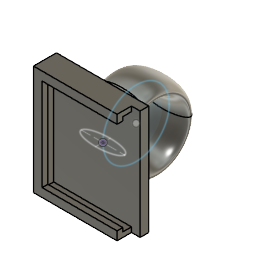
JoystickRingM1 (Autodesk Fusion 360 design; units mm, degrees)
part number: 2026-01-29-20-05-59-741
Autodesk Fusion 360 part; units mm, degrees
sketch "Sketch1" plane through (0, 0, 0) normal (0, 0, 1) x (1, 0, 0)
  ellipse E0 centre (0, 0) end of major axis (7.5, 0) minor radius 2.5
  line L0 (-7.5, 0) -> (7.5, 0) construction
  line L1 (0, -2.5) -> (0, 2.5) construction
  dimension "d1" = 15
  dimension "d2" = 5
  constraint coincident E0 L0.start
  constraint coincident E0 L0.end
  constraint coincident E0 L1.start
  constraint coincident E0 L1.end
  constraint coincident E0.centre origin
  constraint horizontal L0
  measures "d1" distance of E0
sketch "Sketch2" plane through (0, 0, 0) normal (1, 0, 0) x (0, 1, 0)
  circle A0 centre (11.5, 0) radius 11.5
  dimension "d4" = 23
  constraint coincident origin A0
  measures "d4" diameter of A0
sweep "Sweep1" add profiles "Sketch1" path "Sketch2" along A0 section 1 makes body 1
sketch "Sketch3" plane through (0, 0, 0) normal (1, 0, 0) x (0, 1, 0)
  line L0 (-0.1, -17.3) -> (-3.1, -17.3)
  line L1 (-3.1, -17.3) -> (-3.1, 17.3)
  line L2 (-3.1, 17.3) -> (-0.1, 17.3)
  line L3 (-0.1, 17.3) -> (-0.1, -17.3)
  dimension "d16" = 34.6
  dimension "d17" = 3
  dimension "d18" = 17.3
  dimension "d19" = 0.1
  constraint horizontal L0
  constraint vertical L1
  constraint horizontal L2
  constraint vertical L3
  measures "d16" distance of L0.start L2.end
  measures "d17" distance of L0.start L0.end
  measures "d18" distance of origin L0
  measures "d19" distance of origin L3
extrude "Extrude1" add sketch "Sketch3" along normal mid plane 28 bodies 1
sketch "Sketch4" plane through (0, -3.1, 0) normal (0, -1, 0) x (1, 0, 0)
  line L0 (-14, -17.3) -> (14, -17.3)
  line L1 (14, -17.3) -> (14, 17.3)
  line L2 (14, 17.3) -> (-14, 17.3)
  line L3 (-14, 17.3) -> (-14, -17.3)
  line L4 (-14, 17.3) -> (-16, 17.3)
  line L5 (-16, 17.3) -> (-16, -17)
  line L6 (-16, -17) -> (-14, -17)
  line L7 (-14, -17) -> (-14, 17.3)
  line L8 (-16, -17) -> (14, -17)
  line L9 (14, -17) -> (14, -19)
  line L10 (14, -19) -> (-16, -19)
  line L11 (-16, -19) -> (-16, -17)
  line L12 (14, -19) -> (16, -19)
  line L13 (16, -19) -> (16, 17)
  line L14 (16, 17) -> (14, 17)
  line L15 (14, 17) -> (14, -19)
  line L16 (16, 17) -> (-16, 17)
  line L17 (-16, 17) -> (-16, 19)
  line L18 (-16, 19) -> (16, 19)
  line L19 (16, 19) -> (16, 17)
  constraint horizontal L4
  constraint vertical L5
  constraint horizontal L6
  constraint vertical L7
  constraint coincident L2.end L3.start
  constraint horizontal L8
  constraint vertical L9
  constraint horizontal L10
  constraint vertical L11
  constraint horizontal L12
  constraint vertical L13
  constraint horizontal L14
  constraint vertical L15
  constraint horizontal L16
  constraint vertical L17
  constraint horizontal L18
  constraint vertical L19
extrude "Extrude2" add sketch "Sketch4" along normal blind 3 separate body contours L0 L3 L6 L8 L9 L10 L11 L15 | L1 L9 L12 L13 L14 L15 L16 | L3 L5 L6 L7 L8 L16 | L3 L4 L5 L7 L16 L17 | L1 L2 L4 L14 L16 L17 L18 L19 makes body 2
sketch "Sketch5" plane through (0, -6.1, 0) normal (0, -1, 0) x (1, 0, 0)
  line L0 (14, -17.3) -> (-14, -17.3)
  line L1 (-14, -17.3) -> (-14, 17.3)
  line L2 (-14, 17.3) -> (14, 17.3)
  line L3 (14, 17.3) -> (14, -17.3)
  line L4 (-16, 19) -> (-16, -19)
  line L5 (-16, -19) -> (16, -19)
  line L6 (16, -19) -> (16, 19)
  line L7 (16, 19) -> (-16, 19)
  line L8 (-16, 19) -> (-13, 19)
  line L9 (-13, 19) -> (-13, -19)
  line L10 (-13, -19) -> (-16, -19)
  line L11 (-16, -19) -> (-16, 19)
  line L12 (-13, -19) -> (16, -19)
  line L13 (16, -19) -> (16, -16)
  line L14 (16, -16) -> (-13, -16)
  line L15 (-13, -16) -> (-13, -19)
  line L16 (16, -19) -> (13, -19)
  line L17 (13, -19) -> (13, 19)
  line L18 (13, 19) -> (16, 19)
  line L19 (16, 19) -> (16, -19)
  line L20 (16, 19) -> (-13, 19)
  line L21 (-13, 19) -> (-13, 16)
  line L22 (-13, 16) -> (16, 16)
  line L23 (16, 16) -> (16, 19)
  constraint horizontal L8
  constraint vertical L9
  constraint horizontal L10
  constraint vertical L11
  constraint coincident L5 L9.end
  constraint coincident L4.start L7.end
  constraint horizontal L12
  constraint vertical L13
  constraint horizontal L14
  constraint vertical L15
  constraint coincident L6 L13.end
  constraint horizontal L16
  constraint vertical L17
  constraint horizontal L18
  constraint vertical L19
  constraint coincident L7 L17.end
  constraint coincident L5.end L6.start
  constraint horizontal L20
  constraint vertical L21
  constraint horizontal L22
  constraint vertical L23
  constraint coincident L9 L21.end
  constraint coincident L6.end L7.start
extrude "Extrude3" add sketch "Sketch5" along normal blind 2 contours L0 L3 L5 L6 L12 L13 L14 L16 L17 L19 | L0 L3 L14 L17 | L0 L5 L9 L12 L15 L17 | L0 L9 L14 L15 L17 | L3 L14 L17 L22 | L3 L6 L14 L19 L22 | L0 L1 L2 L4 L5 L7 L8 L9 L10 L11 L15 L21 | L0 L1 L2 L9 L15 L21 | L2 L3 L17 L22 | L2 L3 L6 L7 L17 L18 L19 L20 L22 L23 | L2 L9 L17 L21 L22 | L2 L7 L9 L17 L20 L21 bodies 2
extrude "Extrude4" add sketch "Sketch4" against normal blind 3 contours L0 L3 L6 L8 L9 L10 L11 L15 | L1 L9 L12 L13 L14 L15 L16 | L3 L5 L6 L7 L8 L16 | L3 L4 L5 L7 L16 L17 | L1 L2 L4 L14 L16 L17 L18 L19 bodies 1 2
sketch "Sketch7" plane through (16, 0, 0) normal (1, 0, 0) x (0, 1, 0)
  line L0 (-0.1, 19) -> (-8.1, 19)
  line L1 (-8.1, 19) -> (-8.1, -19)
  line L2 (-8.1, -19) -> (-0.1, -19)
  line L3 (-0.1, -19) -> (-0.1, 19)
  line L4 (-8.1, 19) -> (-3.1, 19)
  line L5 (-3.1, 19) -> (-3.1, -19)
  line L6 (-3.1, -19) -> (-8.1, -19)
  line L7 (-8.1, -19) -> (-8.1, 19)
  dimension "d34" = 3
  dimension "d35" = 5
  constraint horizontal L4
  constraint vertical L5
  constraint horizontal L6
  constraint vertical L7
  constraint coincident L2 L5.end
  measures "d34" distance of L3 L5
  measures "d35" distance of L5.end L1.end
extrude "Extrude6" cut sketch "Sketch7" against normal blind 3 contours L0 L1 L2 L4 L5 L6 L7 bodies 1
fillet "Fillet1" radius 5 2 edges at (1.4908, -0.1, -7.749) (-1.4908, -0.1, 7.749) on bodies 1
equation "d18 = ( 34.6 / 2 ) * 1 mm"
